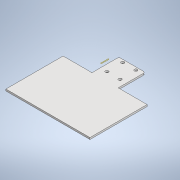
# Autodesk Inventor part: Part9
Saved by Autodesk Inventor 2022 (Build 260153000, 153)
## iProperties
Created: 2022-12-25
Part Number: Part9
Material: ABS Plastic
Document SubType Name: Modeling
Designer: Kamil
Mass: 165.869 g
Surface Area: 155.846 cm^2
Volume: 21.4578 cm^3
Density: 1.06 g/cm^3
Appearance: Smooth - White
Author: Kamil
Autodesk Inventor part; units mm, degrees
ref_plane "YZ Plane" through (0, 0, 0) normal (1, 0, 0) x (0, 1, 0)
ref_plane "XZ Plane" through (0, 0, 0) normal (0, 1, 0) x (-1, 0, 0)
ref_plane "XY Plane" through (0, 0, 0) normal (0, 0, 1) x (1, 0, 0)
ref_plane "Work Plane1" through (41.5591, -8.9669, 74.6916) normal (0, -1, 0) x (-1, 0, 0)
sketch "Sketch1" plane through (41.5591, -8.9669, 74.6916) normal (0, -1, 0) x (-1, 0, 0)
  line L0 (-33.5, 15.2) -> (-33.5, 8.8885) projected
  line L1 (-33.5, 8.8885) -> (-3.5, 8.8885) projected
  line L2 (-3.5, 8.8885) -> (-3.5, 15.2) projected
  arc A0 (-3.5, 15.2) -> (-5.5, 17.2) centre (-5.5, 15.2) ccw projected
  line L3 (-5.5, 17.2) -> (-31.5, 17.2) projected
  arc A1 (-31.5, 17.2) -> (-33.5, 15.2) centre (-31.5, 15.2) ccw projected
  circle A2 centre (-26, 14) radius 1.75 projected
  circle A3 centre (-11, 14) radius 1.75 projected
  line L4 (-14.3359, 1.1115) -> (-14.3359, -7.2) projected
  line L5 (-14.3359, -7.2) -> (-5.5, -7.2) projected
  arc A4 (-5.5, -7.2) -> (-3.5, -5.2) centre (-5.5, -5.2) ccw projected
  line L6 (-3.5, -5.2) -> (-3.5, 1.1115) projected
  line L7 (-3.5, 1.1115) -> (-14.3359, 1.1115) projected
  circle A5 centre (-11, -4) radius 1.75 projected
  line L8 (1, 1) -> (1, 9) projected
  line L9 (1, 9) -> (0, 9) projected
  line L10 (0, 1) -> (0, 9) projected
  line L11 (0, 1) -> (1, 1) projected
  line L12 (3.5, 1) -> (3.5, 9) projected
  line L13 (3.5, 1) -> (4.5, 1) projected
  line L14 (4.5, 1) -> (4.5, 9) projected
  line L15 (4.5, 9) -> (3.5, 9) projected
  circle A6 centre (-26, -4) radius 1.75 projected
  line L16 (-22.6641, -7.2) -> (-22.6641, 1.1115) projected
  line L17 (-22.6641, 1.1115) -> (-33.5, 1.1115) projected
  line L18 (-33.5, 1.1115) -> (-33.5, -5.2) projected
  arc A7 (-33.5, -5.2) -> (-31.5, -7.2) centre (-31.5, -5.2) ccw projected
  line L19 (-31.5, -7.2) -> (-22.6641, -7.2) projected
  line L20 (29.5, -11.1) -> (-1.3, -11.1)
  line L21 (-3.5, -7.2) -> (-33.5, -7.2)
  line L22 (-33.5, -7.2) -> (-33.5, 17.2)
  line L23 (-33.5, 17.2) -> (-3.5, 17.2)
  line L24 (-3.5, 17.2) -> (-3.5, -7.2)
  line L25 (29.5, 21.1) -> (-1.3, 21.1)
  line L26 (29.5, 21.1) -> (31.5, 21.1)
  line L27 (31.5, 21.1) -> (-68.5, 21.1)
  line L28 (-68.5, 21.1) -> (-68.5, -78.9)
  line L29 (-68.5, -78.9) -> (31.5, -78.9)
  line L30 (31.5, -78.9) -> (31.5, 21.1)
  line L31 (-18.5, -78.9) -> (-18.5, 21.1)
  line L32 (29.5, -11.1) -> (-1.3, -11.1)
  line L33 (-1.3, -11.1) -> (-1.3, -13.6)
  line L34 (-1.3, -13.6) -> (29.5, -13.6)
  line L35 (29.5, -13.6) -> (29.5, -11.1)
  line L36 (29.5, -13.6) -> (-18.5, -13.6)
  line L37 (-18.5, -13.6) -> (-18.5, -78.9)
  line L38 (-18.5, -78.9) -> (29.5, -78.9)
  line L39 (29.5, -78.9) -> (29.5, -13.6)
  line L40 (-3.5, -7.2) -> (-18.5, -7.2)
  line L41 (-18.5, -7.2) -> (-18.5, -13.6)
  line L42 (-18.5, -13.6) -> (-3.5, -13.6)
  line L43 (-3.5, -13.6) -> (-3.5, -7.2)
  line L44 (-66.5, -13.6) -> (-18.5, -13.6)
  line L45 (-66.5, -78.9) -> (-66.5, -13.6)
  line L46 (-33.5, -13.6) -> (-33.5, -7.2)
  point P0 (41.5591, 74.6916)
  point P1 (-3.5, 8.8885)
  point P2 (-33.5, 1.1115)
  point P3 (-33.5, -5.2)
  point P4 (-33.5, -13.6)
  point P5 (-66.5, -78.9)
  point P6 (29.5, -78.9)
  point P7 (-1.3, -13.6)
  point P8 (-3.5, -13.6)
  point P9 (-3.5, -5.2)
  point P10 (-3.5, 1.1115)
  dimension "d0" = 2
  dimension "d1" = 100
  dimension "d2" = 100
  dimension "d3" = 2.5
  constraints: 54 end point, 10 parallel, 8 horizontal, 5 perpendicular, 3 symmetric about line, 2 midpoint, 4 other
  measures "d0" distance of L25.start L26.end
  measures "d1" distance of L29.end L28.end
  measures "d2" distance of L28.end L27.end
  measures "d3" distance of L33.end L32.end
extrude "Extrusion1" add sketch "Sketch1" along normal blind 2 contours A1 L3 L31 L1 L0 | L1 L31 L21 L16 L17 L22 | L31 L3 A0 L2 L1 | L1 L24 L7 L4 L21 L31 | L17 L16 L19 A7 L18 | L31 L44 L46 L21 L19 | L21 L5 L43 L36 L31 | A7 L21 L22 | L6 A4 L5 L4 L7 | L36 L34 L39 L29 L31 | L31 L29 L45 L44 | L24 L21 A4
sketch "Sketch2" plane through (41.5591, -10.9669, 74.6916) normal (0, -1, 0) x (1, 0, 0)
  arc A0 (3.5, -15.2) -> (5.5, -17.2) centre (5.5, -15.2) ccw projected
  line L0 (5.5, -17.2) -> (31.5, -17.2) projected
  arc A1 (31.5, -17.2) -> (33.5, -15.2) centre (31.5, -15.2) ccw projected
  line L1 (33.5, -15.2) -> (33.5, 13.6) projected
  line L2 (33.5, 13.6) -> (66.5, 13.6) projected
  line L3 (66.5, 13.6) -> (66.5, 78.9) projected
  line L4 (66.5, 78.9) -> (-29.5, 78.9) projected
  line L5 (-29.5, 78.9) -> (-29.5, 13.6) projected
  line L6 (-29.5, 13.6) -> (3.5, 13.6) projected
  line L7 (3.5, 13.6) -> (3.5, -15.2) projected
  circle A2 centre (26, -14) radius 1.75 projected
  circle A3 centre (26, 4) radius 1.75 projected
  circle A4 centre (11, 4) radius 1.75 projected
  circle A5 centre (11, -14) radius 1.75 projected
  point P0 (-41.5591, -74.6916)
extrude "Extrusion2" add sketch "Sketch2" along normal blind 4.5
sketch "Sketch3" plane through (41.5591, -15.4669, 74.6916) normal (0, -1, 0) x (1, 0, 0)
  line L0 (5.5, -17.2) -> (31.5, -17.2) projected
  arc A0 (31.5, -17.2) -> (33.5, -15.2) centre (31.5, -15.2) ccw projected
  line L1 (33.5, -15.2) -> (33.5, 13.6) projected
  line L2 (33.5, 13.6) -> (66.5, 13.6) projected
  line L3 (66.5, 13.6) -> (66.5, 78.9) projected
  line L4 (66.5, 78.9) -> (-29.5, 78.9) projected
  line L5 (-29.5, 78.9) -> (-29.5, 13.6) projected
  line L6 (-29.5, 13.6) -> (3.5, 13.6) projected
  line L7 (3.5, 13.6) -> (3.5, -15.2) projected
  arc A1 (3.5, -15.2) -> (5.5, -17.2) centre (5.5, -15.2) ccw projected
  circle A2 centre (26, -14) radius 1.75 projected
  circle A3 centre (26, 4) radius 1.75 projected
  circle A4 centre (11, 4) radius 1.75 projected
  circle A5 centre (11, -14) radius 1.75 projected
  point P0 (-41.5591, -74.6916)
extrude "Extrusion3" add sketch "Sketch3" along normal blind 1.1
sketch "Sketch4" plane through (41.5591, -8.9669, 74.6916) normal (0, 1, 0) x (1, 0, 0)
  arc A0 (5.5, 17.2) -> (3.5, 15.2) centre (5.5, 15.2) ccw projected
  line L0 (3.5, -13.6) -> (3.5, 15.2) projected
  line L1 (-29.5, -13.6) -> (3.5, -13.6) projected
  line L2 (-29.5, -78.9) -> (-29.5, -13.6) projected
  line L3 (66.5, -78.9) -> (-29.5, -78.9) projected
  line L4 (66.5, -13.6) -> (66.5, -78.9) projected
  line L5 (33.5, -13.6) -> (66.5, -13.6) projected
  line L6 (33.5, 15.2) -> (33.5, -13.6) projected
  arc A1 (33.5, 15.2) -> (31.5, 17.2) centre (31.5, 15.2) ccw projected
  line L7 (5.5, 17.2) -> (31.5, 17.2) projected
  circle A2 centre (26, 14) radius 1.75 projected
  circle A3 centre (26, -4) radius 1.75 projected
  circle A4 centre (11, -4) radius 1.75 projected
  circle A5 centre (11, 14) radius 1.75 projected
  point P0 (-41.5591, 74.6916)
extrude "Extrusion4" cut sketch "Sketch4" against normal blind 4.6
sketch "Sketch5" plane through (41.5591, -13.5669, 74.6916) normal (0, 1, 0) x (1, 0, 0)
  line L0 (5.5, 17.2) -> (31.5, 17.2) projected
  arc A0 (5.5, 17.2) -> (3.5, 15.2) centre (5.5, 15.2) ccw projected
  line L1 (3.5, -13.6) -> (3.5, 15.2) projected
  line L2 (-29.5, -13.6) -> (3.5, -13.6) projected
  line L3 (-29.5, -78.9) -> (-29.5, -13.6) projected
  line L4 (66.5, -78.9) -> (-29.5, -78.9) projected
  line L5 (66.5, -13.6) -> (66.5, -78.9) projected
  line L6 (33.5, -13.6) -> (66.5, -13.6) projected
  line L7 (33.5, 15.2) -> (33.5, -13.6) projected
  arc A1 (33.5, 15.2) -> (31.5, 17.2) centre (31.5, 15.2) ccw projected
  circle A2 centre (11, 14) radius 1.75 projected
  circle A3 centre (11, -4) radius 1.75 projected
  circle A4 centre (26, -4) radius 1.75 projected
  circle A5 centre (26, 14) radius 1.75 projected
  point P0 (-41.5591, 74.6916)
extrude "Extrusion5" add sketch "Sketch5" along normal blind 0.1
sketch "Sketch6" plane through (41.5591, -16.5669, 74.6916) normal (0, -1, 0) x (1, 0, 0)
  arc A0 (31.5, -17.2) -> (33.5, -15.2) centre (31.5, -15.2) ccw projected
  line L0 (33.5, -15.2) -> (33.5, 13.6) projected
  line L1 (33.5, 13.6) -> (66.5, 13.6) projected
  line L2 (66.5, 13.6) -> (66.5, 78.9) projected
  line L3 (66.5, 78.9) -> (-29.5, 78.9) projected
  line L4 (-29.5, 78.9) -> (-29.5, 13.6) projected
  line L5 (-29.5, 13.6) -> (3.5, 13.6) projected
  line L6 (3.5, 13.6) -> (3.5, -15.2) projected
  arc A1 (3.5, -15.2) -> (5.5, -17.2) centre (5.5, -15.2) ccw projected
  line L7 (5.5, -17.2) -> (31.5, -17.2) projected
  circle A2 centre (26, -14) radius 1.75 projected
  circle A3 centre (26, 4) radius 1.75 projected
  circle A4 centre (11, 4) radius 1.75 projected
  circle A5 centre (11, -14) radius 1.75 projected
  point P0 (-41.5591, -74.6916)
extrude "Extrusion6" cut sketch "Sketch6" against normal blind 0.1
sketch "Sketch7" plane through (41.5591, -13.4669, 74.6916) normal (0, 1, 0) x (1, 0, 0)
  line L0 (31.5, 17.2) -> (5.5, 17.2) projected
  arc A0 (5.5, 17.2) -> (3.5, 15.2) centre (5.5, 15.2) ccw projected
  line L1 (3.5, 15.2) -> (3.5, -13.6) projected
  line L2 (3.5, -13.6) -> (-29.5, -13.6) projected
  line L3 (-29.5, -13.6) -> (-29.5, -78.9) projected
  line L4 (-29.5, -78.9) -> (66.5, -78.9) projected
  line L5 (66.5, -78.9) -> (66.5, -13.6) projected
  line L6 (66.5, -13.6) -> (33.5, -13.6) projected
  line L7 (33.5, -13.6) -> (33.5, 15.2) projected
  arc A1 (33.5, 15.2) -> (31.5, 17.2) centre (31.5, 15.2) ccw projected
  circle A2 centre (11, 14) radius 1.75 projected
  circle A3 centre (11, -4) radius 1.75 projected
  circle A4 centre (26, -4) radius 1.75 projected
  circle A5 centre (26, 14) radius 1.75 projected
  circle A6 centre (18.5, 5) radius 2.6186 projected
  arc A7 (3.5, -5.2) -> (5.5, -7.2) centre (5.5, -5.2) ccw projected
  line L8 (9.1525, -7.2) -> (5.5, -7.2) projected
  line L9 (7.305, -4) -> (9.1525, -7.2) projected
  line L10 (9.1525, -0.8) -> (7.305, -4) projected
  line L11 (12.8475, -0.8) -> (9.1525, -0.8) projected
  line L12 (14.695, -4) -> (12.8475, -0.8) projected
  line L13 (12.8475, -7.2) -> (14.695, -4) projected
  line L14 (24.1525, -7.2) -> (12.8475, -7.2) projected
  line L15 (24.1525, -7.2) -> (22.305, -4) projected
  line L16 (22.305, -4) -> (24.1525, -0.8) projected
  line L17 (24.1525, -0.8) -> (27.8475, -0.8) projected
  line L18 (27.8475, -0.8) -> (29.695, -4) projected
  line L19 (29.695, -4) -> (27.8475, -7.2) projected
  line L20 (27.8475, -7.2) -> (31.5, -7.2) projected
  arc A8 (31.5, -7.2) -> (33.5, -5.2) centre (31.5, -5.2) ccw projected
  line L21 (33.5, -5.2) -> (33.5, 15.2) projected
  arc A9 (33.5, 15.2) -> (31.5, 17.2) centre (31.5, 15.2) ccw projected
  line L22 (31.5, 17.2) -> (27.8475, 17.2) projected
  line L23 (27.8475, 17.2) -> (29.695, 14) projected
  line L24 (29.695, 14) -> (27.8475, 10.8) projected
  line L25 (27.8475, 10.8) -> (24.1525, 10.8) projected
  line L26 (24.1525, 10.8) -> (22.305, 14) projected
  line L27 (22.305, 14) -> (24.1525, 17.2) projected
  line L28 (24.1525, 17.2) -> (12.8475, 17.2) projected
  line L29 (14.695, 14) -> (12.8475, 17.2) projected
  line L30 (12.8475, 10.8) -> (14.695, 14) projected
  line L31 (9.1525, 10.8) -> (12.8475, 10.8) projected
  line L32 (7.305, 14) -> (9.1525, 10.8) projected
  line L33 (9.1525, 17.2) -> (7.305, 14) projected
  line L34 (5.5, 17.2) -> (9.1525, 17.2) projected
  arc A10 (5.5, 17.2) -> (3.5, 15.2) centre (5.5, 15.2) ccw projected
  line L35 (3.5, -5.2) -> (3.5, 15.2) projected
  line L36 (12.8475, -7.2) -> (9.1525, -7.2) projected
  line L37 (24.1525, -7.2) -> (27.8475, -7.2) projected
  line L38 (66.5, -13.6) -> (33.5, -13.6) projected
  line L39 (3.5, -13.6) -> (33.5, -13.6)
  point P0 (-41.5591, 74.6916)
  constraints: 2 end point, 1 collinear
extrude "Extrusion7" add sketch "Sketch7" along normal blind 4.5 contours A1 L7 A8 L20 L19 L18 L17 L16 L15 L14 L13 L12 L11 L10 L9 L8 A7 L1 A0 L0 L33 L32 L31 L30 L29 L27 L26 L25 L24 L23 | L23 L24 L25 L26 L27 L0 | L7 L39 L1 A7 L8 L36 L14 L37 L20 A8 | L29 L30 L31 L32 L33 L0 | L37 L15 L16 L17 L18 L19 | L36 L9 L10 L11 L12 L13 | A6
sketch "Sketch8" plane through (41.5591, -13.4669, 74.6916) normal (0, 1, 0) x (1, 0, 0)
  line L0 (33.5, -13.6) -> (3.5, -13.6) projected
  line L1 (3.5, -13.6) -> (-29.5, -13.6) projected
  line L2 (-29.5, -13.6) -> (-29.5, -78.9) projected
  line L3 (-29.5, -78.9) -> (66.5, -78.9) projected
  line L4 (66.5, -78.9) -> (66.5, -13.6) projected
  line L5 (66.5, -13.6) -> (33.5, -13.6) projected
  point P0 (-41.5591, 74.6916)
extrude "Extrusion8" add sketch "Sketch8" along normal blind 4.5
sketch "Sketch9" plane through (41.5591, -16.4669, 74.6916) normal (0, -1, 0) x (1, 0, 0)
  line L0 (33.5, 13.6) -> (33.5, -15.2) projected
  line L1 (66.5, 13.6) -> (33.5, 13.6) projected
  line L2 (66.5, 78.9) -> (66.5, 13.6) projected
  line L3 (-29.5, 78.9) -> (66.5, 78.9) projected
  line L4 (-29.5, 13.6) -> (-29.5, 78.9) projected
  line L5 (3.5, 13.6) -> (-29.5, 13.6) projected
  line L6 (3.5, -15.2) -> (3.5, 13.6) projected
  arc A0 (3.5, -15.2) -> (5.5, -17.2) centre (5.5, -15.2) ccw projected
  line L7 (31.5, -17.2) -> (5.5, -17.2) projected
  arc A1 (31.5, -17.2) -> (33.5, -15.2) centre (31.5, -15.2) ccw projected
  circle A2 centre (26, -14) radius 1.75 projected
  circle A3 centre (26, 4) radius 1.75 projected
  circle A4 centre (11, 4) radius 1.75 projected
  circle A5 centre (11, -14) radius 1.75 projected
  point P0 (-41.5591, -74.6916)
extrude "Extrusion9" cut sketch "Sketch9" against normal blind 0.4
sketch "Sketch10" plane through (41.5591, -16.0669, 74.6916) normal (0, -1, 0) x (1, 0, 0)
  line L0 (31.5, -17.2) -> (5.5, -17.2) projected
  arc A0 (31.5, -17.2) -> (33.5, -15.2) centre (31.5, -15.2) ccw projected
  line L1 (33.5, 13.6) -> (33.5, -15.2) projected
  line L2 (66.5, 13.6) -> (33.5, 13.6) projected
  line L3 (66.5, 78.9) -> (66.5, 13.6) projected
  line L4 (-29.5, 78.9) -> (66.5, 78.9) projected
  line L5 (-29.5, 13.6) -> (-29.5, 78.9) projected
  line L6 (3.5, 13.6) -> (-29.5, 13.6) projected
  line L7 (3.5, -15.2) -> (3.5, 13.6) projected
  arc A1 (3.5, -15.2) -> (5.5, -17.2) centre (5.5, -15.2) ccw projected
  circle A2 centre (26, -14) radius 1.75 projected
  circle A3 centre (26, 4) radius 1.75 projected
  circle A4 centre (11, 4) radius 1.75 projected
  circle A5 centre (11, -14) radius 1.75 projected
  line L8 (-29.5, 78.9) -> (66.5, 78.9) projected
  line L9 (-29.5, 13.6) -> (-29.5, 78.9) projected
  line L10 (66.5, 78.9) -> (-29.5, 78.9)
  line L11 (-29.5, 78.9) -> (-29.5, 75.9)
  line L12 (-29.5, 75.9) -> (66.5, 75.9)
  line L13 (66.5, 75.9) -> (66.5, 78.9)
  line L14 (3.5, 13.6) -> (-29.5, 13.6) projected
  line L15 (-29.5, 78.9) -> (-26.5, 78.9)
  line L16 (-26.5, 78.9) -> (-26.5, 13.6)
  line L17 (-26.5, 13.6) -> (-29.5, 13.6)
  line L18 (-29.5, 13.6) -> (-29.5, 78.9)
  line L19 (66.5, 13.6) -> (33.5, 13.6) projected
  line L20 (66.5, 75.9) -> (63.5, 75.9)
  line L21 (63.5, 75.9) -> (63.5, 13.6)
  line L22 (63.5, 13.6) -> (66.5, 13.6)
  line L23 (66.5, 13.6) -> (66.5, 75.9)
  point P0 (-41.5591, -74.6916)
  point P1 (63.5, 75.9)
  point P2 (-26.5, 75.9)
  point P3 (-26.5, 13.6)
  dimension "d22" = 3
  dimension "d23" = 3
  dimension "d24" = 3
  constraints: 24 end point, 6 parallel, 3 horizontal, 3 perpendicular, 3 point on line
  measures "d22" distance of L11.end L10.end
  measures "d23" distance of L16.end L17.end
  measures "d24" distance of L22.end L21.end
extrude "Extrusion10" cut sketch "Sketch10" against normal blind 1.5 contours L0 A1 L7 L6 L16 L12 L21 L2 L1 A0
sketch "Sketch11" plane through (41.5591, -14.5669, 74.6916) normal (0, -1, 0) x (1, 0, 0)
  arc A0 (3.5, -15.2) -> (5.5, -17.2) centre (5.5, -15.2) ccw projected
  line L0 (31.5, -17.2) -> (5.5, -17.2) projected
  arc A1 (31.5, -17.2) -> (33.5, -15.2) centre (31.5, -15.2) ccw projected
  line L1 (33.5, 13.6) -> (33.5, -15.2) projected
  line L2 (63.5, 13.6) -> (33.5, 13.6) projected
  line L3 (63.5, 75.9) -> (63.5, 13.6) projected
  line L4 (-26.5, 75.9) -> (63.5, 75.9) projected
  line L5 (-26.5, 13.6) -> (-26.5, 75.9) projected
  line L6 (3.5, 13.6) -> (-26.5, 13.6) projected
  line L7 (3.5, -15.2) -> (3.5, 13.6) projected
  circle A2 centre (26, -14) radius 1.75 projected
  circle A3 centre (26, 4) radius 1.75 projected
  circle A4 centre (11, 4) radius 1.75 projected
  circle A5 centre (11, -14) radius 1.75 projected
  line L8 (-26.5, 13.6) -> (-26.5, 75.9) projected
  line L9 (-26.5, 44.75) -> (63.5, 44.75)
  point P0 (-41.5591, -74.6916)
  point P1 (-26.5, 44.75)
  constraints: 2 end point, 2 midpoint
extrude "Extrusion11" cut sketch "Sketch11" against normal blind 1.5 contours L7 L6 L5 L9 L3 L2 L1 A1 L0 A0
sketch "Sketch12" plane through (41.5591, -14.5669, 74.6916) normal (0, -1, 0) x (1, 0, 0)
  line L0 (-26.5, 44.75) -> (63.5, 44.75) projected
  circle A0 centre (11, -14) radius 1.75 projected
  circle A1 centre (11, 4) radius 1.75 projected
  circle A2 centre (26, 4) radius 1.75 projected
  circle A3 centre (26, -14) radius 1.75 projected
  line L1 (14, -17.2) -> (14, -0.0594) projected
  line L2 (14, -0.0594) -> (23, -0.0594) projected
  line L3 (23, -0.0594) -> (23, -17.2) projected
  line L4 (23, -17.2) -> (31.5, -17.2) projected
  arc A4 (31.5, -17.2) -> (33.5, -15.2) centre (31.5, -15.2) ccw projected
  line L5 (33.5, -15.2) -> (33.5, 13.6) projected
  line L6 (33.5, 13.6) -> (63.5, 13.6) projected
  line L7 (63.5, 13.6) -> (63.5, 75.9) projected
  line L8 (63.5, 75.9) -> (-26.5, 75.9) projected
  line L9 (-26.5, 75.9) -> (-26.5, 13.6) projected
  line L10 (-26.5, 13.6) -> (3.5, 13.6) projected
  line L11 (3.5, 13.6) -> (3.5, -15.2) projected
  arc A5 (3.5, -15.2) -> (5.5, -17.2) centre (5.5, -15.2) ccw projected
  line L12 (5.5, -17.2) -> (14, -17.2) projected
  point P0 (-41.5591, -74.6916)
extrude "Extrusion12" cut sketch "Sketch12" against normal blind 1.5 contours L9 L8 L7 L0
sketch "Sketch13" plane through (41.5591, -13.0669, 74.6916) normal (0, -1, 0) x (1, 0, 0)
  line L0 (3.5, -15.2) -> (3.5, 13.6) projected
  arc A0 (3.5, -15.2) -> (5.5, -17.2) centre (5.5, -15.2) ccw projected
  line L1 (31.5, -17.2) -> (5.5, -17.2) projected
  arc A1 (31.5, -17.2) -> (33.5, -15.2) centre (31.5, -15.2) ccw projected
  line L2 (33.5, 13.6) -> (33.5, -15.2) projected
  line L3 (63.5, 13.6) -> (33.5, 13.6) projected
  line L4 (63.5, 75.9) -> (63.5, 13.6) projected
  line L5 (-26.5, 75.9) -> (63.5, 75.9) projected
  line L6 (-26.5, 13.6) -> (-26.5, 75.9) projected
  line L7 (3.5, 13.6) -> (-26.5, 13.6) projected
  circle A2 centre (26, -14) radius 1.75 projected
  circle A3 centre (26, 4) radius 1.75 projected
  circle A4 centre (11, 4) radius 1.75 projected
  circle A5 centre (11, -14) radius 1.75 projected
  point P0 (-41.5591, -74.6916)
extrude "Extrusion13" add sketch "Sketch13" along normal blind 1
sketch "Sketch14" plane through (41.5591, -14.0669, 74.6916) normal (0, -1, 0) x (1, 0, 0)
  circle A0 centre (18.5, -5) radius 2.6186 projected
  line L0 (33.5, -15.2) -> (33.5, 13.6) projected
  line L1 (33.5, 13.6) -> (63.5, 13.6) projected
  line L2 (63.5, 75.9) -> (63.5, 13.6) projected
  line L3 (-26.5, 75.9) -> (63.5, 75.9) projected
  line L4 (-26.5, 13.6) -> (-26.5, 75.9) projected
  line L5 (-26.5, 13.6) -> (3.5, 13.6) projected
  line L6 (3.5, 13.6) -> (3.5, -15.2) projected
  arc A1 (3.5, -15.2) -> (5.5, -17.2) centre (5.5, -15.2) ccw projected
  line L7 (5.5, -17.2) -> (31.5, -17.2) projected
  arc A2 (31.5, -17.2) -> (33.5, -15.2) centre (31.5, -15.2) ccw projected
  circle A3 centre (26, -14) radius 1.75 projected
  circle A4 centre (26, 4) radius 1.75 projected
  circle A5 centre (11, 4) radius 1.75 projected
  circle A6 centre (11, -14) radius 1.75 projected
  line L8 (31.5, -17.2) -> (5.5, -17.2) projected
  line L9 (18.5, 0.1885) -> (23, 0.1885)
  line L10 (23, 0.1885) -> (23, -17.2)
  line L11 (23, -17.2) -> (18.5, -17.2)
  line L12 (18.5, -17.2) -> (18.5, 0.1885)
  line L13 (18.5, 0.1885) -> (14, 0.1885)
  line L14 (14, 0.1885) -> (14, -17.2)
  line L15 (14, -17.2) -> (18.5, -17.2)
  line L16 (18.5, -17.2) -> (18.5, 0.1885)
  point P0 (-41.5591, -74.6916)
  point P1 (23, -17.2)
  point P2 (14, -17.2)
  dimension "d33" = 4.5
  dimension "d34" = 4.5
  constraints: 16 end point, 4 parallel, 2 horizontal, 2 perpendicular, 2 point on line
  measures "d33" distance of L10.end L11.end
  measures "d34" distance of L15.end L14.end
extrude "Extrusion14" cut sketch "Sketch14" against normal blind 1 contours A0 L12 | A0 L12 L9 L10 L7 | L12 A0 | A0 L12 L7 L14 L13
sketch "Sketch15" plane through (41.5591, -13.0669, 74.6916) normal (0, -1, 0) x (1, 0, 0)
  circle A0 centre (18.5, -5) radius 2.6186 projected
  point P0 (-41.5591, -74.6916)
extrude "Extrusion15" cut sketch "Sketch15" against normal through all
sketch "Sketch16" plane through (108.0591, -8.9669, 153.5916) normal (1, 0, 0) x (0, 0, -1)
  circle A0 centre (83.9, 6) radius 16.1 projected
  line L0 (0, -7.1) -> (65.3, -7.1) projected
  line L1 (65.3, 0) -> (65.3, -7.1) projected
  line L2 (0, 0) -> (65.3, 0) projected
  line L3 (0, 0) -> (0, -7.1) projected
  line L4 (83.9, -10.1) -> (0, -10.1)
  line L5 (0.8502, -10.1) -> (13.5781, 2.6279)
  line L6 (13.5781, 2.6279) -> (15.6995, 0.5066)
  line L7 (15.6995, 0.5066) -> (5.0929, -10.1)
  point P0 (153.5916, 8.9669)
  point P1 (8.0929, -7.1)
  point P2 (15.1929, 0)
  dimension "d39" = 18
  dimension "d40" = 45
  dimension "d41" = 3
  constraints: 8 end point, 2 horizontal, 2 point on line, 1 perpendicular, 1 vertical alignment, 1 other
  measures "d39" distance of L5.start L5.end
  measures "d40" angle of L4 L5
  measures "d41" distance of L5.end L6.end
extrude "Extrusion16" cut sketch "Sketch16" against normal through all contours L3 L2 L5 L0 | L5 L2 L7 L0
sketch "Sketch17" plane through (108.0591, -16.0669, 88.2916) normal (1, 0, 0) x (0, 0, -1)
  line L0 (-49.6005, 11.8492) -> (-64.4498, -3) projected
  line L1 (-64.4498, -3) -> (-60.2071, -3) projected
  line L2 (-60.2071, -3) -> (-47.4792, 9.7279) projected
  line L3 (-47.4792, 9.7279) -> (-49.6005, 11.8492) projected
  line L4 (-50.1071, 7.1) -> (-57.2071, 0) projected
  line L5 (-57.2071, 0) -> (0, 0) projected
  line L6 (0, 7.1) -> (0, 0) projected
  line L7 (-50.1071, 7.1) -> (0, 7.1) projected
  line L8 (-47.4792, 9.7279) -> (-13.2443, 43.9628)
  line L9 (-47.4792, 9.7279) -> (-48.8934, 11.1421)
  line L10 (-48.8934, 11.1421) -> (-14.6585, 45.377)
  line L11 (-14.6585, 45.377) -> (-13.2443, 43.9628)
  circle A0 centre (18.6, 13.1) radius 16.1 projected
  line L12 (0, 7.1) -> (0, 18.2927)
  circle A1 centre (18.6, 13.1) radius 18.6
  line L13 (18.6, 29.2) -> (18.6, 35.2)
  line L14 (18.6, 35.2) -> (-22.0071, 35.2)
  point P0 (88.2916, 16.0669)
  point P1 (0, 13.1)
  point P2 (18.6, 31.7)
  dimension "d44" = 2
  dimension "d45" = 6
  constraints: 14 end point, 3 point on line, 2 perpendicular, 2 vertical, 1 centre point, 1 coincident, 1 parallel, 1 tangent, 1 vertical alignment, 1 other
  measures "d44" distance of L2.end L9.end
  measures "d45" distance of L13.start L13.end
extrude "Extrusion17" add sketch "Sketch17" against normal blind 5 contours L8 L14 L13 A1 L12 L7 L2
sketch "Sketch18" plane through (12.0591, -16.0669, 88.2916) normal (-1, 0, 0) x (0, 0, 1)
  line L0 (50.1071, 7.1) -> (22.0071, 35.2) projected
  line L1 (22.0071, 35.2) -> (-18.6, 35.2) projected
  line L2 (-18.6, 35.2) -> (-18.6, 31.7) projected
  arc A0 (0, 13.1) -> (-18.6, 31.7) centre (-18.6, 13.1) ccw projected
  line L3 (0, 13.1) -> (0, 7.1) projected
  line L4 (50.1071, 7.1) -> (0, 7.1) projected
  point P0 (-88.2916, 16.0669)
extrude "Extrusion18" add sketch "Sketch18" against normal blind 5
sketch "Sketch19" plane through (12.0591, -16.0669, 88.2916) normal (-1, 0, 0) x (0, 0, 1)
  line L0 (57.2071, 0) -> (22.0071, 35.2) projected
  line L1 (22.0071, 35.2) -> (-18.6, 35.2) projected
  line L2 (-18.6, 35.2) -> (-18.6, 31.7) projected
  arc A0 (0, 13.1) -> (-18.6, 31.7) centre (-18.6, 13.1) ccw projected
  line L3 (0, 13.1) -> (0, 0) projected
  line L4 (0, 0) -> (57.2071, 0) projected
  point P0 (-88.2916, 16.0669)
extrude "Extrusion19" add sketch "Sketch19" along normal blind 1.5
sketch "Sketch20" plane through (108.0591, -16.0669, 145.4987) normal (1, 0, 0) x (0, 0, -1)
  line L0 (35.2, 35.2) -> (0, 0) projected
  line L1 (0, 0) -> (57.2071, 0) projected
  line L2 (57.2071, 13.1) -> (57.2071, 0) projected
  arc A0 (75.8071, 31.7) -> (57.2071, 13.1) centre (75.8071, 13.1) ccw projected
  line L3 (75.8071, 31.7) -> (75.8071, 35.2) projected
  line L4 (75.8071, 35.2) -> (35.2, 35.2) projected
  point P0 (145.4987, 16.0669)
extrude "Extrusion20" add sketch "Sketch20" along normal blind 1.5
sketch "Sketch21" plane through (103.0591, 15.6331, 69.6916) normal (0, 0, -1) x (-1, 0, 0)
  line L0 (0, 0) -> (-6.5, 0) projected
  line L1 (0, 0) -> (-6.5, 0) projected
  line L2 (0, 3.5) -> (0, 0) projected
  line L3 (0, 3.5) -> (-6.5, 3.5) projected
  line L4 (-6.5, 0) -> (-6.5, 3.5) projected
  line L5 (86, 3.5) -> (92.5, 3.5) projected
  line L6 (86, 0) -> (86, 3.5) projected
  line L7 (86, 0) -> (92.5, 0) projected
  line L8 (92.5, 3.5) -> (92.5, 0) projected
  point P0 (103.0591, -15.6331)
  point P1 (-6.5, 0)
ref_plane "Work Plane2" through (47.0591, -8.4669, 57.4916) normal (0, 0, -1) x (0, 1, 0)
extrude "Extrusion21" add sketch "Sketch21" along normal up to surface (12.2 mm away)
sketch "Sketch22" plane through (15.0591, -14.0669, 143.4987) normal (0, 0.7071068, 0.7071068) x (1, 0, 0)
  line L0 (0, 0) -> (0, -2.8284) projected
  line L1 (90, 0) -> (0, 0) projected
  line L2 (90, -2.8284) -> (90, 0) projected
  line L3 (94.5, -2.8284) -> (90, -2.8284) projected
  line L4 (94.5, 46.9519) -> (94.5, -2.8284) projected
  line L5 (94.5, 46.9519) -> (88, 46.9519) projected
  line L6 (88, 7.2125) -> (88, 46.9519) projected
  line L7 (2, 7.2125) -> (88, 7.2125) projected
  line L8 (2, 46.9519) -> (2, 7.2125) projected
  line L9 (2, 46.9519) -> (-4.5, 46.9519) projected
  line L10 (-4.5, -2.8284) -> (-4.5, 46.9519) projected
  line L11 (0, -2.8284) -> (-4.5, -2.8284) projected
  line L12 (2, 7.2125) -> (88, 7.2125) projected
  line L13 (90, 0) -> (0, 0) projected
  line L14 (2, 7.2125) -> (88, 7.2125)
  line L15 (88, 7.2125) -> (88, 0)
  line L16 (88, 0) -> (2, 0)
  line L17 (2, 0) -> (2, 7.2125)
  line L18 (45, 7.2125) -> (45, 0)
  line L19 (2, 3.6062) -> (88, 3.6062)
  circle A0 centre (25.1488, 4.642) radius 1.5
  circle A1 centre (64.8512, 4.642) radius 1.5
  point P0 (-15.0591, 111.4157)
  dimension "d56" = 3
  constraints: 12 end point, 4 midpoint, 2 centre point, 2 parallel, 1 horizontal, 1 perpendicular, 1 point on line, 1 symmetric about line, 1 other
  measures "d56" diameter of A0
extrude "Extrusion22" cut sketch "Sketch22" against normal blind 10 contours A0 L19 | L19 A0 | A1 L19 | L19 A1
ref_plane "Work Plane3" through (15.0591, -16.5417, 141.0239) normal (0, 0.7071068, 0.7071068) x (1, 0, 0)
sketch "Sketch23" plane through (15.0591, -16.5417, 141.0239) normal (0, 0.7071068, 0.7071068) x (1, 0, 0)
  circle A0 centre (64.8512, 4.642) radius 1.5 projected
  circle A1 centre (25.1488, 4.642) radius 1.5 projected
  line L0 (90, -1.4142) -> (0, -1.4142) projected
  line L1 (64.8512, -1.4142) -> (68.9404, -1.4142)
  line L2 (68.9404, -1.4142) -> (68.9404, 8.1917)
  line L3 (68.9404, 8.1917) -> (64.8512, 8.1917)
  line L4 (64.8512, 8.1917) -> (64.8512, -1.4142)
  line L5 (60.7619, -1.4142) -> (60.7619, 8.1917)
  line L6 (60.7619, 8.1917) -> (64.8512, 8.1917)
  line L7 (90, 0) -> (0, 0) projected
  line L8 (45, 0) -> (45, 11.0699)
  line L9 (21.0596, -1.4142) -> (21.0596, 8.1917)
  line L10 (21.0596, 8.1917) -> (25.1488, 8.1917)
  line L11 (29.2381, -1.4142) -> (29.2381, 8.1917)
  line L12 (29.2381, 8.1917) -> (25.1488, 8.1917)
  point P0 (-15.0591, 111.4157)
  point P1 (21.0596, -1.4142)
  point P2 (29.2381, -1.4142)
  point P3 (64.8512, 3.142)
  point P4 (64.8512, 6.142)
  point P5 (60.7619, -1.4142)
  point P6 (68.9404, -1.4142)
  constraints: 22 end point, 7 symmetric about line, 2 parallel, 1 horizontal, 1 midpoint, 1 perpendicular, 1 point on line, 1 vertical
extrude "Extrusion23" cut sketch "Sketch23" against normal blind 10 contours A0 L4 | A0 L4 L3 L2 L7 | A0 L4 L7 L5 L6 | L7 L2 L0 L4 | L4 L0 L5 L7 | L0 L9 L7 L11 | L7 L9 L10 L12 L11 picked at (65.676, 4.9537)
sketch "Sketch24" plane through (109.5591, -16.0669, 145.4987) normal (1, 0, 0) x (0, 0, -1)
  line L0 (35.2, 35.2) -> (88.0071, 35.2) projected
  line L1 (35.2, 35.2) -> (0, 0) projected
  line L2 (0, 0) -> (57.2071, 0) projected
  line L3 (57.2071, 0) -> (57.2071, 13.1) projected
  arc A0 (75.8071, 31.7) -> (57.2071, 13.1) centre (75.8071, 13.1) ccw projected
  line L4 (75.8071, 31.7) -> (88.0071, 31.7) projected
  line L5 (88.0071, 31.7) -> (88.0071, 35.2) projected
  line L6 (88.0071, 31.7) -> (88.0071, 35.2) projected
  line L7 (88.0071, 31.7) -> (91.0071, 31.7)
  line L8 (91.0071, 31.7) -> (91.0071, 35.2)
  line L9 (91.0071, 35.2) -> (88.0071, 35.2)
  line L10 (88.0071, 35.2) -> (88.0071, 31.7)
  line L11 (91.0071, 35.2) -> (35.2, 35.2)
  line L12 (35.2, 35.2) -> (35.2, 40.2)
  line L13 (35.2, 40.2) -> (91.0071, 40.2)
  line L14 (91.0071, 40.2) -> (91.0071, 35.2)
  line L15 (35.2, 35.2) -> (40.2, 40.2)
  point P0 (145.4987, 16.0669)
  dimension "d62" = 3
  dimension "d63" = 5
  constraints: 18 end point, 4 parallel, 2 horizontal, 2 perpendicular, 1 point on line
  measures "d62" distance of L9.end L8.end
  measures "d63" distance of L11.end L12.end
extrude "Extrusion24" add sketch "Sketch24" against normal up to surface (6.5 mm away) contours L15 L13 L14 L9 L0 | L9 L8 L7 L5
sketch "Sketch25" plane through (10.5591, -16.0669, 88.2916) normal (-1, 0, 0) x (0, 0, 1)
  line L0 (0, 0) -> (57.2071, 0) projected
  line L1 (57.2071, 0) -> (22.0071, 35.2) projected
  line L2 (22.0071, 35.2) -> (-30.8, 35.2) projected
  line L3 (-30.8, 35.2) -> (-30.8, 31.7) projected
  line L4 (-18.6, 31.7) -> (-30.8, 31.7) projected
  arc A0 (0, 13.1) -> (-18.6, 31.7) centre (-18.6, 13.1) ccw projected
  line L5 (0, 13.1) -> (0, 0) projected
  line L6 (50.1071, 7.1) -> (17.0071, 40.2) projected
  line L7 (17.0071, 40.2) -> (-33.8, 40.2) projected
  line L8 (-33.8, 40.2) -> (-33.8, 31.7) projected
  line L9 (-18.6, 31.7) -> (-33.8, 31.7) projected
  arc A1 (0, 13.1) -> (-18.6, 31.7) centre (-18.6, 13.1) ccw projected
  line L10 (0, 13.1) -> (0, 7.1) projected
  line L11 (50.1071, 7.1) -> (0, 7.1) projected
  point P0 (-88.2916, 16.0669)
extrude "Extrusion25" add sketch "Sketch25" against normal up to surface (6.5 mm away) contours L2 L3 L9 L8 L7 L6
body "Solid1"
